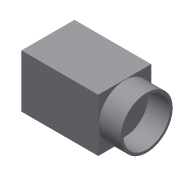
# Autodesk Inventor part: 00_Basler_acA1920_25gm
Saved by Autodesk Inventor 2019 (Build 230136000, 136)
## iProperties
Created: 2019-10-23
Part Number: 00_Basler_acA1920_25gm
Material: Generic
Document SubType Name: Modeling
Designer: diederichbenedict
Density: 1 g/cm^3
Appearance: Default
Author: diederichbenedict
Autodesk Inventor part; units mm, degrees
ref_plane "YZ Plane" through (0, 0, 0) normal (1, 0, 0) x (0, 1, 0)
ref_plane "XZ Plane" through (0, 0, 0) normal (0, 1, 0) x (-1, 0, 0)
ref_plane "XY Plane" through (0, 0, 0) normal (0, 0, 1) x (1, 0, 0)
sketch "Sketch1" plane through (0, 0, 0) normal (0, 0, 1) x (1, 0, 0)
  line L0 (0, 0) -> (42, 0)
  line L1 (42, 0) -> (42, 29)
  line L2 (42, 29) -> (0, 29)
  line L3 (0, 29) -> (0, 0)
  dimension "d0" = 42
  dimension "d1" = 29
  constraints: 8 end point, 2 parallel, 1 horizontal, 1 perpendicular
  measures "d0" distance of L2.end L1.end
  measures "d1" distance of L1.end L0.end
extrude "Extrusion1" add sketch "Sketch1" along normal blind 29
sketch "Sketch2" plane through (42, 0, 0) normal (1, 0, 0) x (0, 0, -1)
  line L0 (0, 0) -> (0, 29) projected
  line L1 (0, 29) -> (-29, 29) projected
  line L2 (-29, 0) -> (-29, 29) projected
  line L3 (0, 0) -> (-29, 0) projected
  circle A0 centre (-14.5, 14.5) radius 14.2
  circle A1 centre (-14.5, 14.5) radius 12.7369
  dimension "d4" = 28.4
  constraints: 2 centre point, 1 coincident
  measures "d4" diameter of A0
extrude "Extrusion2" add sketch "Sketch2" along normal blind 12 contours A0
sketch "Sketch3" plane through (0, 0, 0) normal (-1, 0, 0) x (0, 0, 1)
  line L0 (0, 29) -> (0, 0) projected
  line L1 (0, 0) -> (29, 0) projected
  line L2 (29, 29) -> (29, 0) projected
  line L3 (0, 29) -> (29, 29) projected
  circle A0 centre (14.5, 14.5) radius 14.2 projected
  circle A1 centre (4.4212, 4.4971) radius 4
  dimension "d7" = 8
  constraints: 1 centre point, 2 other
  measures "d7" diameter of A1
extrude "Extrusion3" add sketch "Sketch3" along normal blind 8 contours A1 A0 | A0 A1 picked at (5.4383, 5.4228) picked at (3.5046, 3.5874)
sketch "Sketch4" plane through (0, 0, 0) normal (0, -1, 0) x (1, 0, 0)
  line L0 (0, 0) -> (42, 0) projected
  line L1 (42, 0) -> (42, 29) projected
  line L2 (0, 29) -> (42, 29) projected
  line L3 (0, 0) -> (0, 29) projected
  line L4 (54, 0.3) -> (54, 28.7) projected
  line L5 (42, 28.7) -> (42, 0.3) projected
  line L6 (54, 14.5) -> (0, 14.5) construction
  line L7 (0, 0) -> (0, 29) construction
  point P0 (38.8, 4.5)
  point P1 (38.8, 24.5)
  point P2 (15.3, 14.5)
  dimension "d10" = 10
  dimension "d11" = 14.5
  dimension "d12" = 3.2
  dimension "d13" = 10
  dimension "d14" = 3.2
  dimension "d15" = 23.5
  constraints: 2 end point, 2 midpoint, 1 horizontal, 1 point on line
  measures "d10" distance from line of point (38.8, 24.5) L6
  measures "d11" distance between parallel lines of L2 L6
  measures "d12" distance from line of point (38.8, 24.5) L1
  measures "d13" distance from line of point (38.8, 4.5) L6
  measures "d14" distance from line of point (38.8, 4.5) L1
  measures "d15" horizontal distance of point (15.3, 14.5) point (38.8, 4.5)
hole "Hole1" at (38.8, 0, 4.5) at (38.8, 0, 24.5) at (15.3, 0, 14.5) direction (0, 1, 0) diameter 2.8 depth 12 tip angle 118
body "Solid1"
